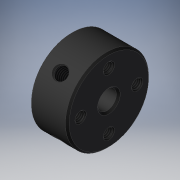
# Autodesk Inventor part: SCMW5b
Saved by Autodesk Inventor 2019 (Build 230136000, 136)
## iProperties
Created: 2022-10-18
Part Number: SCMW5b
Material: Generic
Catalog Web Link: www.cadenas.de
Description: SCMW, PSCMW, SSCMW_b-Shaft Collars - Set Screw, with 4 Holes
Vendor: MISUMI
Document SubType Name: Modeling
Designer: psAdmin
Manufacturer: MISUMI
Mass: 3.24332 g
Surface Area: 19.2101 cm^2
Volume: 3.24332 cm^3
Density: 1 g/cm^3
Appearance: PSOLRGB-175-175-175
Category: PARTsolutions
Company: MISUMI
Title: SCMW5
Author: Cadenas PARTsolutions
Comments: Shaft Collars - Set Screw, with 4 Holes
PSOL_IDENT_0: {$CADENAS_DATA/23d-libs/misumi/metric/03_set_collars/scmw/scmw_b.prj},171 {VTYP=3D},{NB=SCMW5b},{LIN
PSOL_IDENT_1: A=SCMW5},{NN=SCMW, PSCMW, SSCMW_b},{DATE=02.06.2021 02:59:54},{GEOMDATE=25.12.2015 06:30:12},{VERSIO
PSOL_IDENT_2: N=},{LINEID=30},{WBVAR=MAT,ST},{WBNUMERIC=}  {NB=SCMW5b},{LINA=SCMW5},{KT=DUMMY},{PN=SCMW5},{TYPE=SC
PSOL_IDENT_3: MW},{MAT=1045},{ST=Black Oxide},{AC=Set Screws 2 Pcs.},{D=5},{B=10},{D1=22},{P=15},{M=M4x4},{THMD=4}
PSOL_IDENT_4: ,{THDMIN=3.242},{M1=M3},{M1NDM=3},{C=0.5},{ST0='Black Oxide','Black Oxide','Electroless Nickel Plati
PSOL_IDENT_5: ng','Electroless Nickel Plating'},{L=4}
NB: SCMW5b
NN: SCMW, PSCMW, SSCMW_b
NT: Shaft Collars - Set Screw, with 4 Holes
NBSYN: $PN.b
LINA: SCMW5
CATALOG: Misumi
PN: SCMW5
MAT: 1045 Carbon Steel Equivalent
ST: Black Oxide
AC: Set Screws 2 Pcs.
D: 5
B: 10
D1: 22
P: 15
M: M4x4
M1: M3
SUPPLIER: MISUMI
ARTICLENO: SCMW5b
BOMINFO: SCMW5
CREATOR: CADENAS GmbH
Autodesk Inventor part; units mm, degrees
sketch "Sketch_1" plane through (0, 0, 0) normal (0, 0, 1) x (1, 0, 0)
  line L0 (0, 0) -> (-5, 0)
  line L1 (-5, 3) -> (-4.5, 2.5)
  line L2 (-4.5, 2.5) -> (4.5, 2.5)
  line L3 (4.5, 2.5) -> (5, 3)
  line L4 (5, 3) -> (5, 10.5)
  line L5 (5, 10.5) -> (4.5, 11)
  line L6 (4.5, 11) -> (-4.5, 11)
  line L7 (-4.5, 11) -> (-5, 10.5)
  line L8 (-5, 10.5) -> (-5, 3)
  constraints: 18 end point
revolve "Revolution1" add sketch "Sketch_1" angle 360 about axis through (0, 0, 0) along (1, 0, 0)
sketch "Sketch_2" plane through (0, 0, 0) normal (1, 0, 0) x (0, 1, 0)
  line L0 (8.556, 8.556) -> (0.9899, 0.9899)
  line L1 (0.9899, 0.9899) -> (-0.4243, 2.4042)
  line L2 (-0.4243, 2.4042) -> (0.3536, 3.182)
  line L3 (0.3536, 3.182) -> (0.8895, 3.182)
  line L4 (0.8895, 3.182) -> (6.364, 8.6564)
  line L5 (6.364, 8.6564) -> (6.364, 9.1924)
  line L6 (6.364, 9.1924) -> (7.1418, 9.9702)
  line L7 (7.1418, 9.9702) -> (8.556, 8.556)
  line L8 (8.556, 8.556) -> (0.9899, 0.9899)
  constraints: 18 end point
revolve "Revolution2" cut sketch "Sketch_2" angle 360 about axis through (0, 8.556, 8.556) along (0, 0.7071, 0.7071)
thread "Thread1" size "M4x0.7" class "6H" standard "ISO Metric profile" full length
sketch "Sketch_3" plane through (0, 0, 0) normal (1, 0, 0) x (0, 1, 0)
  line L0 (-8.556, 8.556) -> (-0.9899, 0.9899)
  line L1 (-0.9899, 0.9899) -> (-2.4042, -0.4243)
  line L2 (-2.4042, -0.4243) -> (-3.182, 0.3536)
  line L3 (-3.182, 0.3536) -> (-3.182, 0.8895)
  line L4 (-3.182, 0.8895) -> (-8.6564, 6.364)
  line L5 (-8.6564, 6.364) -> (-9.1924, 6.364)
  line L6 (-9.1924, 6.364) -> (-9.9702, 7.1418)
  line L7 (-9.9702, 7.1418) -> (-8.556, 8.556)
  line L8 (-8.556, 8.556) -> (-0.9899, 0.9899)
  constraints: 18 end point
revolve "Revolution3" cut sketch "Sketch_3" angle 360 about axis through (0, -8.556, 8.556) along (0, -0.7071, 0.7071)
thread "Thread2" size "M4x0.7" class "6H" standard "ISO Metric profile" full length
sketch "Sketch_10" plane through (0, 0, 0) normal (0, 1, 0) x (-1, 0, 0)
  line L0 (-5, -7.5) -> (5, -7.5)
  line L1 (5, -7.5) -> (5, -9)
  line L2 (5, -9) -> (4.7295, -8.7295)
  line L3 (4.7295, -8.7295) -> (-4.7295, -8.7295)
  line L4 (-4.7295, -8.7295) -> (-5, -9)
  line L5 (-5, -9) -> (-5, -7.5)
  line L6 (-5, -7.5) -> (5, -7.5)
  constraints: 14 end point
revolve "Revolution4" cut sketch "Sketch_10" angle 360 about axis through (5, 0, -7.5) along (1, 0, 0)
thread "Thread3" size "M3x0.5" class "6H" standard "ISO Metric profile" full length
sketch "Sketch_11" plane through (0, 0, 0) normal (0, 1, 0) x (-1, 0, 0)
  line L0 (-5, 7.5) -> (5, 7.5)
  line L1 (5, 7.5) -> (5, 6)
  line L2 (5, 6) -> (4.7295, 6.2705)
  line L3 (4.7295, 6.2705) -> (-4.7295, 6.2705)
  line L4 (-4.7295, 6.2705) -> (-5, 6)
  line L5 (-5, 6) -> (-5, 7.5)
  line L6 (-5, 7.5) -> (5, 7.5)
  constraints: 14 end point
revolve "Revolution5" cut sketch "Sketch_11" angle 360 about axis through (5, 0, 7.5) along (1, 0, 0)
thread "Thread4" size "M3x0.5" class "6H" standard "ISO Metric profile" full length
sketch "Sketch_12" plane through (0, 0, 0) normal (0, 0, 1) x (1, 0, 0)
  line L0 (5, 7.5) -> (-5, 7.5)
  line L1 (-5, 7.5) -> (-5, 9)
  line L2 (-5, 9) -> (-4.7295, 8.7295)
  line L3 (-4.7295, 8.7295) -> (4.7295, 8.7295)
  line L4 (4.7295, 8.7295) -> (5, 9)
  line L5 (5, 9) -> (5, 7.5)
  line L6 (5, 7.5) -> (-5, 7.5)
  constraints: 14 end point
revolve "Revolution6" cut sketch "Sketch_12" angle 360 about axis through (5, 7.5, 0) along (1, 0, 0)
thread "Thread5" size "M3x0.5" class "6H" standard "ISO Metric profile" full length
sketch "Sketch_13" plane through (0, 0, 0) normal (0, 0, 1) x (1, 0, 0)
  line L0 (5, -7.5) -> (-5, -7.5)
  line L1 (-5, -7.5) -> (-5, -6)
  line L2 (-5, -6) -> (-4.7295, -6.2705)
  line L3 (-4.7295, -6.2705) -> (4.7295, -6.2705)
  line L4 (4.7295, -6.2705) -> (5, -6)
  line L5 (5, -6) -> (5, -7.5)
  line L6 (5, -7.5) -> (-5, -7.5)
  constraints: 14 end point
revolve "Revolution7" cut sketch "Sketch_13" angle 360 about axis through (5, -7.5, 0) along (1, 0, 0)
thread "Thread6" size "M3x0.5" class "6H" standard "ISO Metric profile" full length
ref_plane "body_set_h_XY" through (0, -7.7782, 7.7782) normal (0, 0.7071, -0.7071) x (1, 0, 0)
ref_plane "body_set_h_YZ" through (0, -7.7782, 7.7782) normal (1, 0, 0) x (0, -0.7071, -0.7071)
ref_plane "body_set_h_ZX" through (0, -7.7782, 7.7782) normal (0, -0.7071, -0.7071) x (0, 0.7071, -0.7071)
ref_plane "body_set_v_XY" through (0, 7.7782, 7.7782) normal (0, 0.7071, 0.7071) x (1, 0, 0)
ref_plane "body_set_v_YZ" through (0, 7.7782, 7.7782) normal (1, 0, 0) x (0, 0.7071, -0.7071)
ref_plane "body_set_v_ZX" through (0, 7.7782, 7.7782) normal (0, 0.7071, -0.7071) x (0, 0.7071, 0.7071)
body "Solid1"
